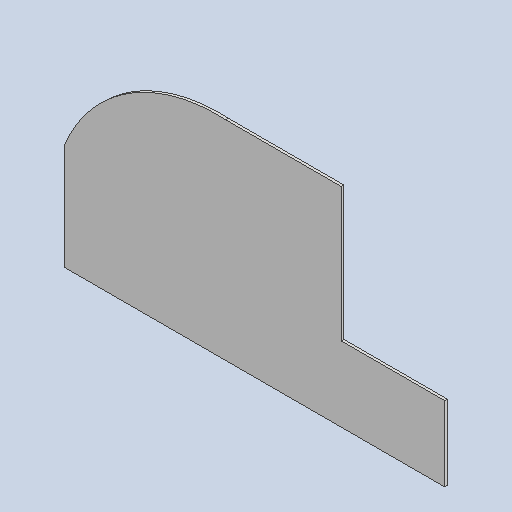
# Autodesk Inventor part: 사이드 카울
Saved by Autodesk Inventor 2025.2 (Build 292293000, 293)
## iProperties
Created: 2025-07-11
Part Number: 사이드 카울
Material: 일반
Document SubType Name: Modeling
Designer: jbhma
Density: 1 g/cm^3
Appearance: 기본값
Author: jbhma
Autodesk Inventor part; units mm, degrees
ref_plane "YZ Plane" through (0, 0, 0) normal (1, 0, 0) x (0, 1, 0)
ref_plane "XZ Plane" through (0, 0, 0) normal (0, 1, 0) x (-1, 0, 0)
ref_plane "XY Plane" through (0, 0, 0) normal (0, 0, 1) x (1, 0, 0)
sketch "스케치1" plane through (0, 0, 0) normal (0, 0, 1) x (1, 0, 0)
  line L0 (552.9734, 795) -> (1055, 795)
  line L1 (1450, 285) -> (1450, 0)
  line L2 (1450, 0) -> (0, 0)
  line L3 (0, 0) -> (0, 405)
  line L4 (0, 0) -> (0, 405) construction
  arc A0 (614, 795) -> (0, 405) centre (583.4867, 164.7107) ccw
  line L5 (1450, 285) -> (1055, 285)
  line L6 (1055, 0) -> (1450, 0)
  line L7 (1450, 0) -> (1450, 285)
  line L8 (1055, 285) -> (1055, 795)
  dimension "d0" = 1450
  dimension "d2" = 405
  dimension "d3" = 631.0275
  dimension "d4" = 836
  dimension "d7" = 285
  dimension "d9" = 395
  dimension "d10" = 510
  dimension "d11" = 395
  constraints: 18 end point, 4 parallel, 3 point on circle, 2 horizontal, 2 perpendicular, 2 point on line, 1 centre point, 1 coincident
  measures "d0" distance of L1.end L2.end
  measures "d2" distance of L3.end L2.end
  measures "d3" radius of A0
  measures "d4" distance from line of A0.start L1
  measures "d7" distance between parallel lines of L2 L5
  measures "d9" distance between parallel lines of L8 L1
  measures "d10" distance between parallel lines of L5 L0
  measures "d11" distance from line of L6.start L1
extrude "돌출1" add sketch "스케치1" along normal blind 10
